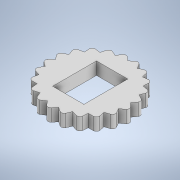
# Autodesk Inventor part: modelGateGear
Saved by Autodesk Inventor 2020 (Build 240168000, 168)
## iProperties
Created: 2023-11-04
Part Number: modelGateGear
Material: Generic
Document SubType Name: Sheet Metal
Designer: jirka
Density: 1 g/cm^3
Sheet Metal Rule: Default_mm
Appearance: Default
Author: jirka
Autodesk Inventor part; units mm, degrees
ref_plane "YZ Plane" through (0, 0, 0) normal (1, 0, 0) x (0, 1, 0)
ref_plane "XZ Plane" through (0, 0, 0) normal (0, 1, 0) x (-1, 0, 0)
ref_plane "XY Plane" through (0, 0, 0) normal (0, 0, 1) x (1, 0, 0)
sketch "Sketch1" plane through (0, 0, 0) normal (0, 1, 0) x (-1, 0, 0)
  line L0 (-3.5, -3.5) -> (0.1946, -3.5) construction
  arc A0 (-5.4544, -2.5) -> (3.5, 4.8734) centre (0, 0) ccw
  line L1 (0, -6) -> (0, -7)
  line L2 (0, -7) -> (1.3359, -5.4079)
  line L3 (0, -7) -> (2.0783, -7) construction
  line L4 (0, -7) -> (-1.4433, -5.2799)
  line L5 (0, -7) -> (2.2454, -7) construction
  circle A1 centre (0, 0) radius 6
  arc A2 (-0.4195, -6.5) -> (0.4195, -6.5) centre (0, -6.228) ccw
  line L6 (2.5, 3.5) -> (-2.5, 3.5)
  line L7 (-2.5, 3.5) -> (-2.5, -3.5)
  line L8 (-2.5, -3.5) -> (2.5, -3.5)
  line L9 (2.5, -3.5) -> (2.5, 3.5)
  point P0 (-204.25, 70)
  point P1 (-7, 0)
  point P2 (-200.75, 67.5)
  point P3 (-0.8955, -5.9328)
  point P4 (0.8955, -5.9328)
  point P5 (-0.3407, -6.594)
  point P6 (0.3407, -6.594)
  point P7 (3.5, 4.8734)
  point P8 (-5.4544, -2.5)
  dimension "d0" = 1
  dimension "d1" = 50
  dimension "d2" = 130
  dimension "d3" = 0.5
  dimension "d6" = 7
  dimension "d7" = 5
  dimension "d8" = 3.5
  dimension "d9" = 2.5
  constraints: 20 end point, 5 point on circle, 4 horizontal, 2 centre point, 2 equal length, 2 parallel, 2 point on line, 1 coincident, 1 perpendicular, 1 vertical, 3 other
  measures "d0" distance of L1.start L1.end
  measures "d1" angle of L3 L2
  measures "d2" angle of L5 L4
  measures "d3" radius of A2
  measures "d6" distance of L6.end L7.end
  measures "d7" distance of L7.end L8.end
  measures "d8" distance from line of point (0, 0) L8
  measures "d9" distance from line of point (0, 0) L7
extrude "Extrusion1" add sketch "Sketch1" along normal blind 2 contours A0 A1
sketch "Sketch2" plane through (0, 2, 0) normal (0, 1, 0) x (1, 0, 0)
  arc A0 (-5.4544, -2.5) -> (3.5, 4.8734) centre (0, 0) ccw
  line L0 (0, -6) -> (0, -7)
  line L1 (0, -7) -> (1.3359, -5.4079)
  line L2 (0, -7) -> (2.0783, -7) construction
  line L3 (0, -7) -> (-1.4433, -5.2799)
  line L4 (0, -7) -> (2.2454, -7) construction
  circle A1 centre (0, 0) radius 6
  arc A2 (-0.4195, -6.5) -> (0.4195, -6.5) centre (0, -6.228) ccw
  point P0 (-200.75, 67.5)
  point P1 (-0.8955, -5.9328)
  point P2 (0.8955, -5.9328)
  point P3 (-0.3407, -6.594)
  point P4 (0.3407, -6.594)
  point P5 (-0.3407, -6.594)
  point P6 (0.3407, -6.594)
  point P7 (0.8955, -5.9328)
  point P8 (-0.8955, -5.9328)
  dimension "d12" = 1
  dimension "d13" = 50
  dimension "d14" = 130
  dimension "d15" = 0.5
  constraints: 10 end point, 5 point on circle, 2 centre point, 2 equal length, 2 horizontal, 2 point on line, 1 coincident, 1 vertical, 1 vertical alignment, 2 other
  measures "d12" distance of L0.start L0.end
  measures "d13" angle of L2 L1
  measures "d14" angle of L4 L3
  measures "d15" radius of A2
extrude "Extrusion2" add sketch "Sketch2" against normal blind 2 contours L3 A0 L0 A2 | L1 A2 L0 A0
pattern_circular "Circular Pattern1" count 21 over 360 about axis through (0, 0, 0) along (0, 1, 0) of "Extrusion2"
equation "\"d8\" = 0.5 * d6"
equation "\"d9\" = 0.5 * d7"
equation "\"BendRadius\" = Thickness"
equation "\"BendReliefWidth\" = Thickness"
equation "\"BendReliefDepth\" = 0.5 * Thickness"
equation "\"CornerReliefSize\" = 4 * Thickness"
equation "\"MinimumRemnant\" = 2 * Thickness"
equation "\"TransitionRadius\" = BendRadius"
equation "\"JacobiRadiusSize\" = BendRadius"
equation "\"GapSize\" = Thickness"
equation "\"Thickness\" = 0.5"
body "Solid1"
